Autodesk Fusion 360 part; units mm, degrees
note: some values were not read from the file. Set by a fixed rule: which sketch regions a step uses.
(part 2 of 2)
sketch "Sketch4" plane through (0, 0, -0.7) normal (0, 0, -1) x (1, 0, 0) in component "Base"
  circle A0 centre (0, 0) radius 5
  circle A1 centre (0, 0) radius 5.4
  line L0 (-5.4, 0) -> (-5.4, -7.4)
  line L1 (-5.4, -7.4) -> (5.4, -7.4)
  line L2 (5.4, -7.4) -> (5.4, 0)
  circle A2 centre (-4, -6.1) radius 0.75
  circle A3 centre (-4, -6.1) radius 0.4
  line L3 (5.4, -6.1) -> (-5.4, -6.1)
  circle A4 centre (-2, -6.1) radius 0.4
  circle A5 centre (-2, -6.1) radius 0.75
  circle A6 centre (0, -6.1) radius 0.4
  circle A7 centre (0, -6.1) radius 0.75
  circle A8 centre (2, -6.1) radius 0.4
  circle A9 centre (2, -6.1) radius 0.75
  circle A10 centre (4, -6.1) radius 0.4
  circle A11 centre (4, -6.1) radius 0.75
  line L4 (-4.3, -7.4) -> (-3.7, -7.4)
  line L5 (-3.7, -7.4) -> (-3.7, -7.7)
  line L6 (-3.7, -7.7) -> (-4.3, -7.7)
  line L7 (-4.3, -7.7) -> (-4.3, -7.4)
  line L8 (-0.3, -7.4) -> (0.3, -7.4)
  line L9 (0.3, -7.4) -> (0.3, -7.7)
  line L10 (0.3, -7.7) -> (-0.3, -7.7)
  line L11 (-0.3, -7.7) -> (-0.3, -7.4)
  line L12 (1.7, -7.4) -> (2.3, -7.4)
  line L13 (2.3, -7.4) -> (2.3, -7.7)
  line L14 (2.3, -7.7) -> (1.7, -7.7)
  line L15 (1.7, -7.7) -> (1.7, -7.4)
  line L16 (3.7, -7.4) -> (4.3, -7.4)
  line L17 (4.3, -7.4) -> (4.3, -7.7)
  line L18 (4.3, -7.7) -> (3.7, -7.7)
  line L19 (3.7, -7.7) -> (3.7, -7.4)
  line L20 (2, -6.1) -> (2, -7.4)
  line L21 (4, -6.1) -> (4, -7.4)
  line L22 (0, -6.1) -> (0, -7.4)
  line L23 (-2.3, -7.4) -> (-1.7, -7.4)
  line L24 (-1.7, -7.4) -> (-1.7, -7.7)
  line L25 (-1.7, -7.7) -> (-2.3, -7.7)
  line L26 (-2.3, -7.7) -> (-2.3, -7.4)
  line L27 (-4, -6.1) -> (-4, -7.4)
  line L28 (-2, -6.1) -> (-2, -7.4)
  line L29 (-5.1, 3.1) -> (-4.8, 3.1)
  line L30 (-4.8, 3.1) -> (-4.8, 2.15)
  line L31 (-4.8, 2.15) -> (-5.1, 2.15)
  line L32 (-5.1, 2.15) -> (-5.1, 3.1)
  line L33 (0, 0) -> (0, 5.4) construction
  line L34 (5.1, 3.1) -> (4.8, 3.1)
  line L35 (4.8, 2.15) -> (5.1, 2.15)
  line L36 (4.8, 3.1) -> (4.8, 2.15)
  line L37 (5.1, 2.15) -> (5.1, 3.1)
  dimension "d21" = 10.8
  dimension "d22" = 7.4
  dimension "d23" = 1.5
  dimension "d24" = 0.8
  dimension "d25" = 1.3
  dimension "d26" = 1.5
  dimension "d27" = 0.8
  dimension "d28" = 1.5
  dimension "d29" = 0.8
  dimension "d30" = 1.5
  dimension "d31" = 0.8
  dimension "d32" = 1.5
  dimension "d33" = 0.8
  dimension "d34" = 2
  dimension "d35" = 2
  dimension "d36" = 2
  dimension "d37" = 2
  dimension "d38" = 0.6
  dimension "d39" = 0.3
  dimension "d42" = 0.3
  dimension "d43" = 0.6
  dimension "d44" = 0.6
  dimension "d45" = 0.3
  dimension "d46" = 0.6
  dimension "d47" = 0.3
  dimension "d49" = 0.6
  dimension "d50" = 0.3
  dimension "d54" = 10.8
  dimension "d55" = 0.3
  dimension "d56" = 0.95
  dimension "d57" = 10.2
  dimension "d66" = 0
  dimension "d67" = 0
  dimension "d68" = 0
  dimension "d69" = 0
  constraint coincident A0.centre A1.centre
  constraint coincident A1 L0.start
  constraint tangent A1 L0
  constraint vertical L0
  constraint perpendicular L0 L1
  constraint coincident A1 L2.end
  constraint tangent A1 L2
  constraint vertical L2
  constraint concentric A2 A3
  constraint coincident L2 L3.start
  constraint coincident L0 L3.end
  constraint perpendicular L0 L3
  constraint coincident A2.centre L3
  constraint concentric A4 A5
  constraint concentric A6 A7
  constraint concentric A8 A9
  constraint concentric A10 A11
  constraint coincident L3 A6.centre
  constraint midpoint L3 A6.centre
  constraint coincident L3 A4.centre
  constraint coincident L3 A8.centre
  constraint coincident L3 A10.centre
  constraint horizontal L4
  constraint vertical L5
  constraint horizontal L6
  constraint vertical L7
  constraint coincident L1 L4.start
  constraint horizontal L8
  constraint vertical L9
  constraint horizontal L10
  constraint vertical L11
  constraint coincident L1 L8.start
  constraint horizontal L12
  constraint vertical L13
  constraint horizontal L14
  constraint vertical L15
  constraint coincident L1 L12.start
  constraint horizontal L16
  constraint vertical L17
  constraint horizontal L18
  constraint vertical L19
  constraint coincident L1 L16.start
  constraint coincident A8.centre A9.centre
  constraint midpoint L12 L20.end
  constraint coincident A10.centre A11.centre
  constraint midpoint L16 L21.end
  constraint vertical L20
  constraint vertical L21
  constraint coincident A6.centre A7.centre
  constraint midpoint L8 L22.end
  constraint vertical L22
  constraint horizontal L23
  constraint vertical L24
  constraint horizontal L25
  constraint vertical L26
  constraint coincident L1 L23.start
  constraint coincident A2.centre A3.centre
  constraint midpoint L4 L27.end
  constraint coincident A4.centre A5.centre
  constraint midpoint L23 L28.end
  constraint vertical L28
  constraint vertical L27
  constraint horizontal L29
  constraint vertical L30
  constraint horizontal L31
  constraint vertical L32
  constraint coincident A1 L33.end
  constraint vertical L33
  constraint symmetric L29.start L33 L34.start
  constraint symmetric L29.end L33 L34.end
  constraint symmetric L30.end L33 L35.start
  constraint symmetric L31.end L33 L35.end
  measures "d21" diameter of A1
  measures "d22" distance of A0.centre L1
  measures "d23" diameter of A2
  measures "d24" diameter of A3
  measures "d25" distance of L1 L3
  measures "d26" diameter of A5
  measures "d27" diameter of A4
  measures "d28" diameter of A7
  measures "d29" diameter of A6
  measures "d30" diameter of A9
  measures "d31" diameter of A8
  measures "d32" diameter of A11
  measures "d33" diameter of A10
  measures "d34" distance of A4.centre A6.centre
  measures "d35" distance of A2.centre A4.centre
  measures "d36" distance of A6.centre A8.centre
  measures "d37" distance of A8.centre A10.centre
  measures "d38" distance of L5.end L6.end
  measures "d39" distance of L4.end L5.end
  measures "d42" distance of L16.start L18.end
  measures "d43" distance of L17.end L18.end
  measures "d44" distance of L13.end L14.end
  measures "d45" distance of L12.end L13.end
  measures "d46" distance of L9.end L10.end
  measures "d47" distance of L8.end L9.end
  measures "d49" distance of L24.end L25.end
  measures "d50" distance of L23.end L24.end
  measures "d54" distance of L6 L29
  measures "d55" distance of L29.start L29.end
  measures "d56" distance of L29.start L31.end
  measures "d57" distance of L32 L37
extrude "Extrude4" add sketch "Sketch4" along normal blind 0.7 separate body contours A0 | A1 A7 L30 L31 L35 L36 | A1 L2 L3 A7 A9 A11 | A1 L35 L36 | L1 L2 L3 A11 L16 L21 | A1 L0 A2 L3 A5 A7 | L1 L3 A7 A9 L8 L12 L20 L22 | A1 L30 L31 | L1 L3 A5 A7 L8 L22 L23 L28 | L1 L3 A9 A11 L12 L16 L20 L21 | L0 L1 A2 L3 L4 L27 | L1 A2 L3 A5 L4 L23 L27 L28 makes body 2 in component "Base"
extrude "Extrude1'" add sketch "Sketch4" along normal up to surface (0.7 mm away) separate body contours A1 L3 A6 A7 | L3 A6 A7 L22 | L3 A10 A11 L21 | L3 A10 A11 | L3 A6 A7 L22 | L3 A8 A9 | L3 A8 A9 L20 | L3 A10 A11 L21 | L3 A4 A5 L28 | L3 A4 A5 | L3 A8 A9 L20 | A2 A3 L3 L27 | A2 A3 L3 | L3 A4 A5 L28 | A2 A3 L3 L27 makes body 3 at (0.3212, 5.4223, -0.9333) makes body 4 at (-1.2509, 6.1374, -1.1667) makes body 5 at (2.7491, 6.1374, -1.1667) makes body 6 at (-3.2509, 6.1374, -1.1667) makes body 7 at (4.7491, 6.1374, -1.1667) in component "Base"
extrude "Extrude2''" add sketch "Sketch4" along normal up to surface (3.2 mm away) separate body contours A1 L35 L36 | A1 L34 L35 L36 L37 | A1 L30 L31 | A1 L29 L30 L31 L32 | L1 L16 L17 L18 L19 | L1 L8 L9 L10 L11 | L1 L12 L13 L14 L15 | L1 L4 L5 L6 L7 | L1 L23 L24 L25 L26 makes body 8 at (4.1, 7.7, -1.7667) makes body 9 at (-4.1, 7.4, -1.7667) makes body 10 at (1.9, 7.4, -1.7667) makes body 11 at (-4.8, -2.7833, -1.7667) makes body 12 at (-2.1, 7.4, -1.7667) makes body 13 at (-0.1, 7.4, -1.7667) makes body 14 at (5.1, -2.4667, -1.7667) in component "Base"
component "Knob" placed x (1, 0, 0) y (0, 1, 0) z (0, 0, 1) at (0, 0, 0)
component "Base" placed x (1, 0, 0) y (0, 1, 0) z (0, 0, 1) at (0, 0, 0)
named bodies: "Body1 (1)"
